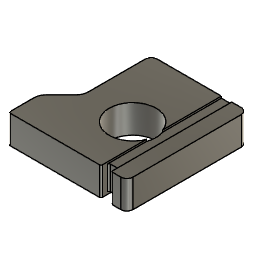
lock_a3 (Autodesk Fusion 360 design; units mm, degrees)
Autodesk Fusion 360 part; units mm, degrees
note: some values were not read from the file. Set by a fixed rule: which sketch regions a step uses.
sketch "Skizze1" plane through (0, 0, 0) normal (0, 0, 1) x (1, 0, 0)
  line L0 (0, 19.86) -> (15.85, 19.86)
  line L1 (15.85, 19.86) -> (15.85, 0)
  circle A0 centre (7.925, 8.925) radius 3.925 construction
  line L2 (-3.65, 5) -> (15.85, 5) construction
  line L3 (4, 19.86) -> (4, 0) construction
  line L4 (0, 0) -> (4, 0)
  line L5 (4, 0) -> (11.57, 0)
  line L6 (11.85, 1.3) -> (13.27, 1.3)
  line L7 (13.27, 1.3) -> (13.27, 0)
  line L8 (13.27, 0) -> (15.85, 0)
  line L9 (11.85, 19.86) -> (11.85, 1.3) construction
  line L10 (11.57, 0) -> (11.57, 1.3)
  line L11 (11.57, 1.3) -> (11.85, 1.3)
  line L12 (11.57, 0) -> (13.27, 0) construction
  line L13 (0, 0) -> (-3.65, 0)
  line L14 (-3.65, 0) -> (-3.65, 5)
  line L15 (-3.65, 5) -> (0, 8.65)
  line L16 (0, 8.65) -> (0, 19.86)
  line L17 (0, 0) -> (0, 8.65) construction
  circle A1 centre (7.925, 8.875) radius 3.875
  line L18 (7.925, 8.875) -> (7.925, 8.925) construction
  dimension "d1" = 7.85
  dimension "d2" = 5
  dimension "d3" = 19.86
  dimension "d4" = 4
  dimension "d5" = 0.28
  dimension "d6" = 1.42
  dimension "d7" = 1.3
  dimension "d8" = 4
  dimension "d9" = 7.65
  dimension "d10" = 5
  dimension "d11" = 135
  dimension "d27" = 7.75
  constraint horizontal L0
  constraint vertical L1
  constraint coincident L1 L2.end
  constraint perpendicular L1 L2
  constraint tangent A0 L2
  constraint coincident L0 L3.start
  constraint tangent A0 L3
  constraint perpendicular L3 L4
  constraint perpendicular L3 L5
  constraint perpendicular L6 L7
  constraint perpendicular L1 L8
  constraint coincident L0 L9.start
  constraint vertical L9
  constraint tangent A0 L9
  constraint horizontal L5
  constraint perpendicular L5 L10
  constraint perpendicular L9 L11
  constraint horizontal L12
  constraint coincident L4.start L13.start
  constraint horizontal L6
  constraint parallel L4 L13
  constraint perpendicular L13 L14
  constraint perpendicular L13 L16
  constraint coincident L2.start L15
  constraint vertical L17
  constraint coincident A1.centre L18.start
  constraint coincident A0.centre L18.end
  constraint vertical L18
  constraint tangent L2 A1
  measures "d1" diameter of A0
  measures "d2" distance of L1.end L2.end
  measures "d3" distance of L0.start L4.start
  measures "d4" distance of L4.start L3.end
  measures "d5" distance of L6.start L10.end
  measures "d6" distance of L6.start L6.end
  measures "d7" distance of L6.end L7.end
  measures "d8" horizontal distance of L1.end L6.start
  measures "d9" distance of L3.end L13.end
  measures "d10" distance of L13.end L2.start
  measures "d11" angle of L14 L15
  measures "d27" diameter of A1
extrude "Extrusion1" add sketch "Skizze1" along normal blind 4.65
sketch "Skizze2" plane through (0, 0, 4.65) normal (0, 0, 1) x (-1, 0, 0)
  line L0 (3.65, 0) -> (-11.57, 0)
  line L1 (-11.57, 0) -> (-11.57, -1.3)
  line L2 (-11.57, -1.3) -> (-13.27, -1.3)
  line L3 (-13.27, -1.3) -> (-13.27, 0)
  line L4 (-13.27, 0) -> (-15.85, 0)
  line L5 (-15.85, 0) -> (-15.85, -19.86)
  line L6 (-15.85, -19.86) -> (0, -19.86)
  line L7 (0, -19.86) -> (0, -8.65)
  line L8 (0, -8.65) -> (3.65, -5)
  line L9 (3.65, -5) -> (3.65, 0)
  line L10 (-11.57, -1.3) -> (-11.57, -19.86)
  line L11 (-11.57, -1.3) -> (-13.27, -1.3)
  line L12 (-13.27, -1.3) -> (-13.27, -19.86)
  line L13 (-13.27, -19.86) -> (-11.57, -19.86)
  circle A0 centre (-7.925, -8.875) radius 3.875
  constraint coincident L1.end L2.start
  constraint coincident L6 L10.end
  constraint perpendicular L6 L10
  constraint coincident L2.end L3.start
  constraint perpendicular L11 L12
  constraint perpendicular L10 L13
extrude "Extrusion2" cut sketch "Skizze2" against normal blind 0.3 contours L2 L6 L10 L11 L12 L13 A0
extrude "Extrusion3" cut sketch "Skizze2" along normal blind 0.4 from surface at -4.65 contours L2 L6 L10 L11 L12 L13 A0
fillet "Abrundung1" radius 1 3 edges at (0, 19.86, 2.325) (15.85, 19.86, 2.325) (15.85, 0, 2.325)
fillet "Abrundung2" radius 0.25 1 edges at (-3.65, 0, 2.325)
fillet "Abrundung3" radius 2 2 edges at (-3.65, 5, 2.325) (0, 8.65, 2.325)
fillet "Abrundung4" radius 0.25 4 edges at (13.27, 0, 2.325) (11.57, 0, 2.325) (11.57, 1.3, 2.375) (13.27, 1.3, 2.375)
equation "d1 = 7.6 mm + 0.25 mm"
equation "d3 = 14 mm + 5.3 mm + 1.2 mm - 0.5 mm - 0.1 mm - 0.04 mm"
